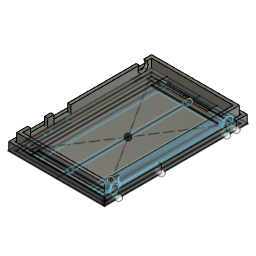
helmet_arduino_case_2_in_1 (Autodesk Fusion 360 design; units mm, degrees)
Autodesk Fusion 360 part; units mm, degrees
note: some values were not read from the file. Set by a fixed rule: which sketch regions a step uses.
sketch "Sketch1" plane through (0, 0, 0) normal (0, 1, 0) x (1, 0, 0) in component "Backer Electronics"
  line L0 (26, 41) -> (-26, 41)
  line L1 (-26, 41) -> (-26, -41)
  line L2 (-26, -41) -> (26, -41)
  line L3 (26, -41) -> (26, 41)
  line L4 (26, 41) -> (-26, -41) construction
  line L5 (-26, 41) -> (26, -41) construction
  line L6 (28, 43) -> (-28, 43)
  line L7 (-28, 43) -> (-28, -43)
  line L8 (-28, -43) -> (28, -43)
  line L9 (28, -43) -> (28, 43)
  line L10 (-21, -36) -> (21, -36)
  line L11 (21, -36) -> (21, 36)
  line L12 (21, 36) -> (-21, 36)
  line L13 (-21, 36) -> (-21, -36)
  line L14 (-26, -36.0289) -> (-28, -36.0289)
  line L15 (-28, -36.0289) -> (-28, -25.2289)
  line L16 (-28, -25.2289) -> (-26, -25.2289)
  line L17 (-26, -25.2289) -> (-26, -36.0289)
  line L18 (-26, -25.2289) -> (-28, -25.2289)
  line L19 (-28, -25.2289) -> (-28, -21.2289)
  line L20 (-28, -21.2289) -> (-26, -21.2289)
  line L21 (-26, -21.2289) -> (-26, -25.2289)
  line L22 (-26, -21.2289) -> (-28, -21.2289)
  line L23 (-28, -21.2289) -> (-28, -10.4289)
  line L24 (-28, -10.4289) -> (-26, -10.4289)
  line L25 (-26, -10.4289) -> (-26, -21.2289)
  line L26 (-21, 36) -> (21, 36)
  line L27 (21, 36) -> (21, 41)
  line L28 (21, 41) -> (-21, 41)
  line L29 (-21, 41) -> (-21, 36)
  line L30 (-21, -36) -> (21, -36)
  line L31 (21, -36) -> (21, -41)
  line L32 (21, -41) -> (-21, -41)
  line L33 (-21, -41) -> (-21, -36)
  line L34 (0, 36) -> (21, 36)
  line L35 (21, 36) -> (21, 41)
  line L36 (21, 41) -> (0, 41)
  line L37 (0, 41) -> (0, 36)
  line L38 (-21, -41) -> (0, -41)
  line L39 (0, -41) -> (0, -36)
  line L40 (0, -36) -> (-21, -36)
  line L41 (-21, -36) -> (-21, -41)
  line L42 (-21, 36) -> (21, 36)
  line L43 (21, 36) -> (21, 36.75)
  line L44 (21, 36.75) -> (-21, 36.75)
  line L45 (-21, 36.75) -> (-21, 36)
  line L46 (-21, -36) -> (21, -36)
  line L47 (21, -36) -> (21, -36.75)
  line L48 (21, -36.75) -> (-21, -36.75)
  line L49 (-21, -36.75) -> (-21, -36)
  circle A0 centre (0, -36.75) radius 1.25
  circle A1 centre (0, 36.75) radius 1.25
  line L50 (-1.25, 36.75) -> (1.25, 36.75)
  line L51 (1.25, 36.75) -> (1.25, -38)
  line L52 (1.25, -38) -> (-1.25, -38)
  line L53 (-1.25, -38) -> (-1.25, 36.75)
  line L54 (1.25, 36.75) -> (-1.25, 36.75)
  line L55 (-1.25, 36.75) -> (-1.25, 41)
  line L56 (-1.25, 41) -> (1.25, 41)
  line L57 (1.25, 41) -> (1.25, 36.75)
  line L58 (-1.25, -36.75) -> (1.25, -36.75)
  line L59 (1.25, -36.75) -> (1.25, -41)
  line L60 (1.25, -41) -> (-1.25, -41)
  line L61 (-1.25, -41) -> (-1.25, -36.75)
  line L62 (-21, -41) -> (-23.5, -41)
  line L63 (-23.5, -41) -> (-23.5, 41)
  line L64 (-23.5, 41) -> (-21, 41)
  line L65 (-21, 41) -> (-21, -41)
  line L66 (21, -41) -> (23.5, -41)
  line L67 (23.5, -41) -> (23.5, 41)
  line L68 (23.5, 41) -> (21, 41)
  line L69 (21, 41) -> (21, -41)
  line L70 (-26, 41) -> (24.577, 41)
  line L71 (24.577, 41) -> (24.577, 38.5)
  line L72 (24.577, 38.5) -> (-26, 38.5)
  line L73 (-26, 38.5) -> (-26, 41)
  line L74 (-26, -41) -> (26, -41)
  line L75 (26, -41) -> (26, -38.5)
  line L76 (26, -38.5) -> (-26, -38.5)
  line L77 (-26, -38.5) -> (-26, -41)
  line L78 (-23.5, -38.5) -> (-18, -38.5)
  line L79 (-18, -38.5) -> (-18, 38.5)
  line L80 (-18, 38.5) -> (-23.5, 38.5)
  line L81 (-23.5, 38.5) -> (-23.5, -38.5)
  line L82 (23.5, -41) -> (18, -41)
  line L83 (18, -41) -> (18, 41)
  line L84 (18, 41) -> (23.5, 41)
  line L85 (23.5, 41) -> (23.5, -41)
  line L86 (-17.9907, -41) -> (-15.4907, -41)
  line L87 (-15.4907, -41) -> (-15.4907, 41)
  line L88 (-15.4907, 41) -> (-17.9907, 41)
  line L89 (-17.9907, 41) -> (-17.9907, -41)
  line L90 (18, -41) -> (15.5, -41)
  line L91 (15.5, -41) -> (15.5, 41)
  line L92 (15.5, 41) -> (18, 41)
  line L93 (18, 41) -> (18, -41)
  dimension "d1" = 52
  dimension "d2" = 82
  dimension "d5" = 2
  dimension "d6" = -5
  dimension "d14" = 10.8
  dimension "d15" = 4
  dimension "d16" = 10.8
  dimension "d22" = 0.75
  dimension "d23" = 0.75
  dimension "d24" = 2.5
  dimension "d25" = 2.5
  dimension "d26" = 2.5
  dimension "d27" = 2.5
  dimension "d28" = 2.5
  dimension "d31" = 2.5
  dimension "d32" = 2.5
  dimension "d33" = 2.5
  dimension "d34" = 2.5
  dimension "d39" = 5.5
  dimension "d40" = 5.5
  dimension "d41" = 2.5
  dimension "d42" = 2.5
  constraint horizontal L0
  constraint perpendicular L0 L1
  constraint parallel L0 L2
  constraint parallel L1 L3
  constraint coincident L4 origin
  constraint coincident L5 origin
  constraint horizontal L14
  constraint vertical L15
  constraint horizontal L16
  constraint vertical L17
  constraint coincident L1 L14.start
  constraint horizontal L18
  constraint vertical L19
  constraint horizontal L20
  constraint vertical L21
  constraint horizontal L22
  constraint vertical L23
  constraint horizontal L24
  constraint vertical L25
  constraint horizontal L26
  constraint vertical L27
  constraint horizontal L28
  constraint vertical L29
  constraint coincident L0 L27.end
  constraint horizontal L30
  constraint vertical L31
  constraint horizontal L32
  constraint vertical L33
  constraint coincident L2 L31.end
  constraint horizontal L34
  constraint vertical L35
  constraint horizontal L36
  constraint vertical L37
  constraint midpoint L26 L34.start
  constraint horizontal L38
  constraint vertical L39
  constraint horizontal L40
  constraint vertical L41
  constraint midpoint L10 L39.end
  constraint horizontal L42
  constraint vertical L43
  constraint horizontal L44
  constraint vertical L45
  constraint horizontal L46
  constraint vertical L47
  constraint horizontal L48
  constraint vertical L49
  constraint midpoint L48 A0.centre
  constraint midpoint L44 A1.centre
  constraint horizontal L50
  constraint vertical L51
  constraint horizontal L52
  constraint vertical L53
  constraint coincident A1 L50.start
  constraint coincident L44 L50.start
  constraint horizontal L54
  constraint vertical L55
  constraint horizontal L56
  constraint vertical L57
  constraint horizontal L58
  constraint vertical L59
  constraint horizontal L60
  constraint vertical L61
  constraint coincident L48 L58.start
  constraint coincident A0 L58.start
  constraint horizontal L62
  constraint vertical L63
  constraint horizontal L64
  constraint vertical L65
  constraint coincident L0 L63.end
  constraint horizontal L66
  constraint vertical L67
  constraint horizontal L68
  constraint vertical L69
  constraint horizontal L70
  constraint vertical L71
  constraint horizontal L72
  constraint vertical L73
  constraint horizontal L74
  constraint vertical L75
  constraint horizontal L76
  constraint vertical L77
  constraint horizontal L78
  constraint vertical L79
  constraint horizontal L80
  constraint vertical L81
  constraint coincident L72 L79.end
  constraint coincident L76 L78.start
  constraint coincident L63 L78.start
  constraint horizontal L82
  constraint vertical L83
  constraint horizontal L84
  constraint vertical L85
  constraint coincident L28 L83.end
  constraint horizontal L86
  constraint vertical L87
  constraint horizontal L88
  constraint vertical L89
  constraint coincident L74 L86.start
  constraint horizontal L90
  constraint vertical L91
  constraint horizontal L92
  constraint vertical L93
  constraint coincident L36 L91.end
  measures "d1" distance of L1.end L2.end
  measures "d2" distance of L0.end L1.end
  measures "d14" distance of L14.start L16.end
  measures "d15" distance of L16.end L20.end
  measures "d16" distance of L20.end L24.end
  measures "d22" distance of L12.end L44.end
  measures "d23" distance of L10.start L48.end
  measures "d24" diameter of A0
  measures "d25" diameter of A1
  measures "d26" distance of L50.start L50.end
  measures "d27" distance of L50.end L50.start
  measures "d28" distance of L58.start L58.end
  measures "d31" distance of L32.end L62.end
  measures "d32" distance of L31.end L66.end
  measures "d33" distance of L0.end L72.end
  measures "d34" distance of L1.end L76.end
  measures "d39" distance of L78.start L78.end
  measures "d40" distance of L66.end L82.end
  measures "d41" distance of L86.start L86.end
  measures "d42" distance of L82.end L90.end
extrude "Extrude6" add sketch "Sketch1" along normal blind 2 contours L1 L7 L20 L22 L23 L24 L25 | L1 L7 L14 L15 L16 L17 L18 makes body 1 at (-26.6667, 0, 32.4289) makes body 2 at (-27.3333, 0, 14.0289) in component "Backer Electronics"
extrude "Extrude2" add sketch "Sketch1" along normal blind 10 separate body contours L0 L1 L2 L3 L6 L7 L8 L9 L14 L24 L28 L32 L36 L38 L56 L60 L62 L64 L66 L68 L70 L73 L74 L75 L77 L82 L84 L86 L88 L90 L92 | L1 L7 L16 L18 L19 L20 L21 L22 makes body 3 at (28, 3.3333, 14.3333) makes body 4 at (-26, 3.3333, 22.5622) in component "Backer Electronics"
extrude "Extrude1" add sketch "Sketch1" along normal blind 1 separate body contours L0 L3 L67 L71 L72 L76 L85 | L0 L67 L70 L71 L72 L85 | L2 L3 L67 L74 L75 L76 L85 | L0 L27 L35 L67 L68 L69 L70 L72 L84 L85 | L2 L31 L66 L67 L69 L74 L76 L82 L85 | L0 L27 L28 L35 L36 L69 L70 L72 L83 L84 L93 | L2 L31 L32 L69 L74 L76 L82 L83 L93 | L0 L28 L36 L70 L72 L83 L91 L92 L93 | L2 L32 L74 L76 L83 L90 L91 L93 | L48 L76 L83 L91 L93 | L0 L28 L36 L57 L70 L72 L91 | L44 L72 L83 L91 L93 | L10 L30 L46 L48 L83 L91 L93 | L2 L32 L59 L74 L76 L91 | L0 L28 L36 L37 L56 L57 L70 L72 | L12 L26 L34 L42 L44 L83 L91 L93 | L10 L12 L26 L30 L34 L42 L46 L83 L91 L93 | L39 L52 L59 L76 | L2 L32 L39 L59 L60 L74 L76 | L0 L28 L37 L55 L56 L70 L72 | L37 A1 L57 L72 | A0 L51 L52 L59 | L10 L30 L46 A0 L51 | L39 L52 L61 L76 | L2 L32 L38 L39 L60 L61 L74 L76 | L0 L28 L55 L70 L72 L87 | L37 A1 L55 L72 | L12 L26 L34 L42 A1 L51 | L10 L12 L26 L30 L34 L40 L42 L46 A0 A1 L51 L53 | A0 L52 L53 L61 | L2 L32 L38 L61 L74 L76 L87 | L0 L28 L70 L72 L87 L88 L89 | L10 L30 L40 L46 A0 L53 | L2 L32 L38 L74 L76 L86 L87 L89 | L48 L76 L87 L89 | L0 L28 L29 L65 L70 L72 L80 L89 | L44 L72 L87 L89 | L12 L26 L42 A1 L53 | L10 L30 L40 L46 L48 L87 L89 | L2 L32 L33 L38 L41 L65 L74 L76 L78 L89 | L0 L29 L63 L64 L65 L70 L72 L80 | L12 L26 L42 L44 L87 L89 | L10 L12 L26 L30 L40 L42 L46 L87 L89 | L0 L1 L63 L70 L72 L73 | L2 L33 L41 L62 L63 L65 L74 L76 L78 | L1 L17 L21 L25 L63 L72 L76 L81 | L1 L2 L63 L74 L76 L77 | L1 L7 L20 L22 L23 L24 L25 | L1 L7 L14 L15 L16 L17 L18 makes body 5 at (-24.3333, 0, 7.0763) in component "Backer Electronics"
extrude "Extrude3" add sketch "Sketch1" along normal blind 4 contours L39 L48 A0 L58 | L10 L30 L39 L46 L48 A0 L58 | L12 L26 L34 L37 L42 L44 A1 L50 L54 | L37 L44 A1 L50 L54 | L10 L30 L39 L40 L46 L48 A0 L58 | L39 L48 A0 L58 | L10 L30 L40 L46 A0 | L37 L44 A1 L50 L54 | L12 L26 L37 L42 L44 A1 L50 L54 | L12 L26 L34 L42 A1 bodies 5 in component "Backer Electronics"
sketch "Sketch1 (1)" plane through (-28, 0, 0) normal (-1, 0, 0) x (0, 0, 1) in component "Backer Electronics"
  line L0 (-43, 0) -> (10.4289, 0)
  line L1 (10.4289, 0) -> (10.4289, 10)
  line L2 (10.4289, 10) -> (-43, 10)
  line L3 (-43, 10) -> (-43, 0)
  line L4 (-38.8228, 10) -> (-32.3228, 10)
  line L5 (-32.3228, 10) -> (-32.3228, 4.5)
  line L6 (-32.3228, 4.5) -> (-38.8228, 4.5)
  line L7 (-38.8228, 4.5) -> (-38.8228, 10)
  line L8 (-38.8228, 4.5) -> (-32.3228, 4.5)
  line L9 (-32.3228, 4.5) -> (-32.3228, 7.75)
  line L10 (-32.3228, 7.75) -> (-38.8228, 7.75)
  line L11 (-38.8228, 7.75) -> (-38.8228, 4.5)
  circle A0 centre (-35.5728, 7.75) radius 3.25
  dimension "d17" = 6.5
  dimension "d18" = 3.25
  dimension "d19" = 6.5
  constraint horizontal L4
  constraint vertical L5
  constraint horizontal L6
  constraint vertical L7
  constraint coincident L2 L4.start
  constraint horizontal L8
  constraint vertical L9
  constraint horizontal L10
  constraint vertical L11
  constraint midpoint L10 A0.centre
  measures "d17" distance of L4.start L4.end
  measures "d18" distance of L6.end L10.end
  measures "d19" diameter of A0
sketch "Sketch2" plane through (28, 0, 0) normal (1, 0, 0) x (0, 0, -1) in component "Backer Electronics"
  line L0 (-43, 0) -> (43, 0)
  line L1 (43, 0) -> (43, 10)
  line L2 (43, 10) -> (-43, 10)
  line L3 (-43, 10) -> (-43, 0)
  circle A0 centre (35.5725, 4.25) radius 3.25
  line L4 (-43, 0) -> (35.5725, 0)
  line L5 (35.5725, 0) -> (35.5725, 4.25)
  line L6 (35.5725, 4.25) -> (-43, 4.25)
  line L7 (-43, 4.25) -> (-43, 0)
  circle A1 centre (-36.2532, 4.25) radius 3.25
  line L8 (-38.9874, 10) -> (-34.0005, 10)
  line L9 (-34.0005, 10) -> (-34.0005, 4.25)
  line L10 (-34.0005, 4.25) -> (-38.9874, 4.25)
  line L11 (-38.9874, 4.25) -> (-38.9874, 10)
  dimension "d20" = 6.5
  dimension "d21" = 6.5
  constraint horizontal L4
  constraint vertical L5
  constraint horizontal L6
  constraint vertical L7
  constraint coincident A0.centre L5.end
  constraint coincident L0.start L3.end
  constraint coincident L6 A1.centre
  constraint horizontal L8
  constraint vertical L9
  constraint horizontal L10
  constraint vertical L11
  constraint coincident L6 L9.end
  constraint coincident L2 L8.start
  measures "d20" diameter of A0
  measures "d21" diameter of A1
extrude "Extrude5" cut sketch "Sketch1 (1)" against normal blind 5 contours L2 L4 L10 A0 | L10 A0 bodies 3 in component "Backer Electronics"
move_face "OffsetFaces1" offset 0.75 1 faces at (-1.25, 0.3333, 12.25) on bodies 5 in component "Backer Electronics"
move_face "OffsetFaces2" offset 0.75 1 faces at (1.25, 0.6667, -12.8333) on bodies 5 in component "Backer Electronics"
sketch "Sketch1 (2)" plane through (0, 0, 0) normal (0, 1, 0) x (1, 0, 0) in component "Lid"
  line L0 (28.5, -43.5) -> (-28.5, -43.5)
  line L1 (-28.5, -43.5) -> (-28.5, 43.5)
  line L2 (-28.5, 43.5) -> (28.5, 43.5)
  line L3 (28.5, 43.5) -> (28.5, -43.5)
  line L4 (28.5, -43.5) -> (-28.5, 43.5) construction
  line L5 (-28.5, -43.5) -> (28.5, 43.5) construction
  line L6 (30.5, 45.5) -> (30.5, -45.5)
  line L7 (30.5, -45.5) -> (-30.5, -45.5)
  line L8 (-30.5, -45.5) -> (-30.5, 45.5)
  line L9 (-30.5, 45.5) -> (30.5, 45.5)
  line L10 (-30.5, 38.4965) -> (-28.5, 38.4965)
  line L11 (-28.5, 38.4965) -> (-28.5, 32.52)
  line L12 (-28.5, 32.52) -> (-30.5, 32.52)
  line L13 (-30.5, 32.52) -> (-30.5, 38.4965)
  line L14 (-30.5, -9.214) -> (-28.5, -9.214)
  line L15 (-28.5, -9.214) -> (-28.5, -36.5)
  line L16 (-28.5, -36.5) -> (-30.5, -36.5)
  line L17 (-30.5, -36.5) -> (-30.5, -9.214)
  line L18 (0, -45.5) -> (0, 45.5)
  line L19 (28.5, 32.52) -> (30.5, 32.52)
  line L20 (30.5, 38.4965) -> (28.5, 38.4965)
  line L21 (30.5, -9.214) -> (28.5, -9.214)
  line L22 (28.5, -36.5) -> (30.5, -36.5)
  line L23 (16, 43.4634) -> (-16, 43.4634)
  line L24 (-16, 43.4634) -> (-16, 34.4634)
  line L25 (-16, 34.4634) -> (16, 34.4634)
  line L26 (16, 34.4634) -> (16, 43.4634)
  line L27 (16, 43.4634) -> (-16, 34.4634) construction
  line L28 (-16, 43.4634) -> (16, 34.4634) construction
  point P0 (0, 38.9634)
  dimension "d45" = 57
  dimension "d46" = 87
  dimension "d47" = -2
  dimension "d52" = 32
  dimension "d53" = 9
  constraint horizontal L0
  constraint perpendicular L0 L1
  constraint parallel L0 L2
  constraint parallel L1 L3
  constraint coincident L4 origin
  constraint coincident L5 origin
  constraint horizontal L10
  constraint vertical L11
  constraint horizontal L12
  constraint vertical L13
  constraint coincident L1 L11.end
  constraint coincident L8 L10.start
  constraint horizontal L14
  constraint vertical L15
  constraint horizontal L16
  constraint vertical L17
  constraint coincident L1 L15.end
  constraint coincident L8 L14.start
  constraint midpoint L7 L18.start
  constraint midpoint L9 L18.end
  constraint symmetric L10.start L18 L20.start
  constraint symmetric L10.end L18 L20.end
  constraint symmetric L11.end L18 L19.start
  constraint symmetric L12.end L18 L19.end
  constraint symmetric L14.start L18 L21.start
  constraint symmetric L14.end L18 L21.end
  constraint symmetric L15.end L18 L22.start
  constraint symmetric L16.end L18 L22.end
  constraint horizontal L23
  constraint perpendicular L23 L24
  constraint parallel L23 L25
  constraint parallel L24 L26
  constraint coincident L27 P0
  constraint coincident L28 P0
  constraint coincident L18 P0
  measures "d45" distance of L1.end L2.end
  measures "d46" distance of L0.end L1.end
  measures "d52" distance of L24.end L25.end
  measures "d53" distance of L23.end L24.end
extrude "Extrude2'" add sketch "Sketch1 (2)" along normal blind 5 separate body contours L0 L3 L6 L7 L18 L22 | L0 L1 L7 L8 L16 L18 | L3 L6 L19 L21 | L1 L8 L14 L15 L16 L17 | L1 L8 L12 L14 | L2 L3 L6 L9 L18 L20 | L1 L2 L8 L9 L10 L18 | L1 L8 L10 L11 L12 L13 makes body 6 at (-30.5, 1.6667, 15.1667) makes body 7 at (28.5, 1.6667, -18.6087) in component "Lid"
extrude "Extrude1'" add sketch "Sketch1 (2)" along normal blind 5 separate body contours L0 L2 L3 L18 L23 L25 L26 | L0 L1 L2 L11 L15 L18 L23 L24 L25 | L3 L6 L21 L22 | L3 L6 L19 L20 makes body 8 in component "Lid"
component "Backer Electronics" placed x (1, 0, 0) y (0, 1, 0) z (0, 0, 1) at (0, 0, 0)
component "Lid" placed x (1, 0, 0) y (0, 1, 0) z (0, 0, 1) at (0, 0, 0)
